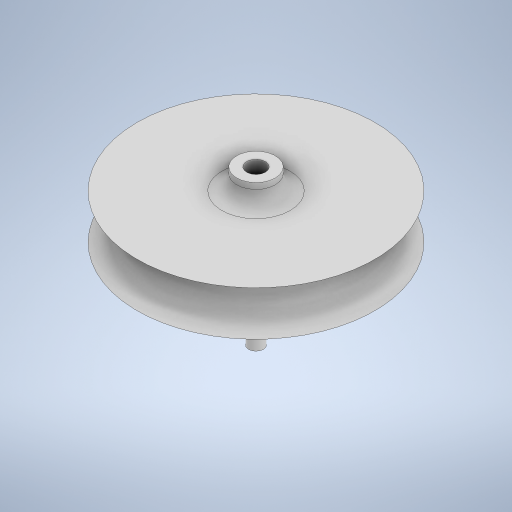
# Autodesk Inventor part: pulley
Saved by Autodesk Inventor 2024 (Build 280153000, 153)
## iProperties
Created: 2024-11-13
Part Number: pulley
Material: Generic
Document SubType Name: Modeling
Designer: manas
Density: 1 g/cm^3
Appearance: Default
Author: manas
Autodesk Inventor part; units mm, degrees
ref_plane "YZ Plane" through (0, 0, 0) normal (1, 0, 0) x (0, 1, 0)
ref_plane "XZ Plane" through (0, 0, 0) normal (0, 1, 0) x (-1, 0, 0)
ref_plane "XY Plane" through (0, 0, 0) normal (0, 0, 1) x (1, 0, 0)
sketch "Sketch1" plane through (0, 0, 0) normal (0, 1, 0) x (-1, 0, 0)
  circle A0 centre (0, 0) radius 40
  dimension "d0" = 80
  constraints: 1 centre point, 1 coincident
  measures "d0" diameter of A0
extrude "Extrusion1" add sketch "Sketch1" along normal blind 15
sketch "Sketch2" plane through (0, 0, 0) normal (1, 0, 0) x (0, 1, 0)
  line L0 (0, 40) -> (15, 40) projected
  line L1 (15, -40) -> (15, 40) projected
  circle A0 centre (7.5, 40) radius 7.5
  point P0 (0, 0)
  constraints: 1 midpoint, 3 other
sketch3d "3D Sketch1"
  arc A0 (-40, 15, 0) -> (0, 15, 40) centre (0, 15, 0) ccw
  arc A1 (0, 15, 40) -> (40, 15, 0) centre (0, 15, 0) ccw
  arc A2 (40, 15, 0) -> (0, 15, -40) centre (0, 15, 0) ccw
  arc A3 (0, 15, -40) -> (-40, 15, 0) centre (0, 15, 0) ccw
sweep "Sweep1" cut profiles "Sketch2" path "3D Sketch1" picked at (7.8013, 37.5182) contours L0 A0
sketch "Sketch3" plane through (0, 15, 0) normal (0, 1, 0) x (1, 0, 0)
  circle A0 centre (0, 0) radius 3.15
  circle A1 centre (0, 0) radius 6.5
  dimension "d5" = 6.3
  dimension "d6" = 13
  constraints: 2 centre point, 2 coincident
  measures "d5" diameter of A0
  measures "d6" diameter of A1
extrude "Extrusion2" add sketch "Sketch3" along normal blind 7
sketch "Sketch4" plane through (0, 0, 0) normal (0, -1, 0) x (1, 0, 0)
  circle A0 centre (0, 0) radius 3.15 projected
  circle A1 centre (0, 0) radius 6.5
  dimension "d9" = 13
  constraints: 1 centre point, 1 coincident
  measures "d9" diameter of A1
extrude "Extrusion3" add sketch "Sketch4" along normal blind 3 contours A0 | A1
sketch "Sketch5" plane through (0, 15, 0) normal (0, 1, 0) x (1, 0, 0)
  circle A0 centre (0, 0) radius 3.15 projected
  circle A1 centre (0, 0) radius 3.15
  dimension "d12" = 6.3
  constraints: 1 centre point, 1 coincident
  measures "d12" diameter of A1
extrude "Extrusion4" cut sketch "Sketch5" against normal blind 15
sketch "Sketch6" plane through (0, -3, 0) normal (0, -1, 0) x (1, 0, 0)
  circle A0 centre (0, 0) radius 3.15 projected
  circle A1 centre (0, 0) radius 2.5
  dimension "d15" = 5
  constraints: 1 centre point, 1 coincident
  measures "d15" diameter of A1
extrude "Extrusion5" add sketch "Sketch6" along normal blind 27 contours A1
fillet "Fillet1" radius 5 1 edges at (-2.5, -3, 0)
fillet "Fillet2" radius 5 1 edges at (-6.5, 0, 0)
fillet "Fillet3" radius 5 1 edges at (-6.5, 15, 0)
body "Solid1"
